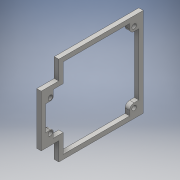
# Autodesk Inventor part: pixy mount front
Saved by Autodesk Inventor 2016 (Build 200138000, 138)
## iProperties
Created: 2015-09-30
Part Number: pixy mount front
Material: Generic
Document SubType Name: Modeling
Designer: Hulbert Office
Density: 1 g/cm^3
Appearance: Default
Author: Hulbert Office
Autodesk Inventor part; units mm, degrees
ref_plane "YZ Plane" through (0, 0, 0) normal (1, 0, 0) x (0, 1, 0)
ref_plane "XZ Plane" through (0, 0, 0) normal (0, 1, 0) x (-1, 0, 0)
ref_plane "XY Plane" through (0, 0, 0) normal (0, 0, 1) x (1, 0, 0)
sketch "Sketch1" plane through (0, 0, 0) normal (1, 0, 0) x (0, 1, 0)
  line L0 (35.3248, 20.4047) -> (35.3248, -21.0933)
  line L1 (29.1498, -27.2683) -> (-15.4752, -27.2683)
  line L2 (-15.4752, -27.2683) -> (-15.4752, -14.5683)
  line L3 (-15.4752, -14.5683) -> (-22.144, -14.5683)
  line L4 (-27.319, -8.7583) -> (-27.319, 8.0697)
  line L5 (-22.144, 13.8797) -> (-15.4752, 13.8797)
  line L6 (-15.4752, 13.8797) -> (-15.4752, 26.5797)
  line L7 (-15.4752, 26.5797) -> (29.1498, 26.5797)
  circle A0 centre (32.1498, 23.4047) radius 1.524
  circle A1 centre (32.1498, -24.0933) radius 1.524
  circle A2 centre (-24.144, -10.7583) radius 1.524
  circle A3 centre (-24.144, 10.0697) radius 1.524
  arc A4 (32.1498, -21.0933) -> (29.1498, -24.0933) centre (32.1498, -24.0933) ccw
  line L8 (29.1498, -24.0933) -> (29.1498, -27.2683)
  line L9 (32.1498, -21.0933) -> (35.3248, -21.0933)
  line L10 (38.3248, -21.0933) -> (38.3248, -27.2683)
  line L11 (38.3248, -27.2683) -> (38.3248, -30.2683)
  line L12 (38.3248, -30.2683) -> (-15.4752, -30.2683)
  line L13 (-15.4752, -30.2683) -> (-18.4752, -30.2683)
  line L14 (-18.4752, -30.2683) -> (-18.4752, -17.8683)
  line L15 (-18.4752, -17.8683) -> (-27.319, -17.8683)
  line L16 (-27.319, -17.8683) -> (-30.319, -17.8683)
  line L17 (-30.319, -17.8683) -> (-30.319, 13.8797)
  line L18 (-30.319, 13.8797) -> (-30.319, 16.8797)
  line L19 (-30.319, 16.8797) -> (-18.4752, 16.8797)
  line L20 (-18.4752, 16.8797) -> (-18.4752, 26.5797)
  line L21 (-18.4752, 26.5797) -> (-18.4752, 29.5797)
  line L22 (-18.4752, 29.5797) -> (35.3248, 29.5797)
  line L23 (35.3248, 29.5797) -> (38.3248, 29.5797)
  line L24 (38.3248, 29.5797) -> (38.3248, -21.0933)
  line L25 (32.1498, 20.4047) -> (38.3248, 20.4047)
  line L26 (29.1498, 23.4047) -> (29.1498, 29.5797)
  arc A5 (29.1498, 23.4047) -> (32.1498, 20.4047) centre (32.1498, 23.4047) ccw
  line L27 (-24.144, 8.0697) -> (-30.319, 8.0697)
  line L28 (-22.144, 10.0697) -> (-22.144, 16.8797)
  arc A6 (-24.144, 8.0697) -> (-22.144, 10.0697) centre (-24.144, 10.0697) ccw
  line L29 (-24.144, -10.7583) -> (-22.144, -10.7583) construction
  line L30 (-24.144, -8.7583) -> (-30.319, -8.7583)
  line L31 (-22.144, -10.7583) -> (-22.144, -17.8683)
  arc A7 (-22.144, -10.7583) -> (-24.144, -8.7583) centre (-24.144, -10.7583) ccw
  line L32 (35.3248, -21.0933) -> (38.3248, -21.0933)
  line L33 (29.1498, -27.2683) -> (29.1498, -30.2683)
  point P0 (0, 0)
  point P1 (0, 0)
  constraints: 68 end point, 20 point on line, 19 perpendicular, 9 point on circle, 8 centre point, 3 horizontal, 2 vertical, 1 collinear, 1 parallel
extrude "Extrusion1" add sketch "Sketch1" along normal blind 3 contours L25 L24 L32 L0 | L25 A5 L26 L22 L23 L24 | L32 L10 L11 L12 L33 L8 A4 L9 | L7 L6 L5 L28 L19 L20 L21 L22 L26 | L33 L12 L13 L14 L15 L31 L3 L2 L1 | L28 A6 L27 L17 L18 L19 | L31 L15 L16 L17 L30 A7 | L4 L30 L17 L27
body "Solid1"
